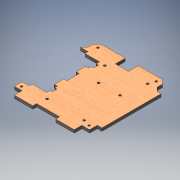
# Autodesk Inventor part: ElectronicPlate
Saved by Autodesk Inventor 2019 (Build 230136000, 136)
## iProperties
Created: 2020-12-31
Part Number: ElectronicPlate
Material: Типовые
Document SubType Name: Modeling
Designer: Professional
Density: 1 g/cm^3
Appearance: Вишневое дерево — натуральный — со слабым глянцем
Author: Professional
Autodesk Inventor part; units mm, degrees
ref_plane "YZ Plane" through (0, 0, 0) normal (1, 0, 0) x (0, 1, 0)
ref_plane "XZ Plane" through (0, 0, 0) normal (0, 1, 0) x (-1, 0, 0)
ref_plane "XY Plane" through (0, 0, 0) normal (0, 0, 1) x (1, 0, 0)
sketch "Эскиз1" plane through (0, 0, 0) normal (0, 1, 0) x (-1, 0, 0)
  line L0 (0, 0) -> (0, -96)
  line L1 (0, 0) -> (15, 0)
  line L2 (15, 0) -> (15, 5)
  line L3 (15, 5) -> (39, 5)
  line L4 (39, 5) -> (39, -5)
  line L5 (39, -5) -> (49, -5)
  line L6 (49, -5) -> (49, -15)
  line L7 (49, -15) -> (55, -15)
  line L8 (55, -15) -> (55, -92)
  line L9 (55, -92) -> (50, -92)
  line L10 (50, -92) -> (45, -97)
  line L11 (45, -97) -> (45, -104)
  line L12 (0, 0) -> (-15, 0)
  line L13 (-15, 0) -> (-15, 5)
  line L14 (-15, 5) -> (-39, 5)
  line L15 (-39, 5) -> (-39, -5)
  line L16 (-39, -5) -> (-49, -5)
  line L17 (-49, -5) -> (-49, -15)
  line L18 (-49, -15) -> (-55, -15)
  line L19 (-55, -15) -> (-55, -92)
  line L20 (-55, -92) -> (-50, -92)
  line L21 (-50, -92) -> (-45, -97)
  line L22 (-45, -97) -> (-45, -104)
  line L23 (45, -104) -> (40, -109)
  line L24 (-40, -109) -> (-45, -104)
  line L25 (40, -109) -> (8.5, -109)
  line L26 (8.5, -109) -> (8.5, -96)
  line L27 (8.5, -96) -> (0, -96)
  line L28 (-40, -109) -> (-8.5, -109)
  line L29 (-8.5, -109) -> (-8.5, -96)
  line L30 (-8.5, -96) -> (0, -96)
  point P0 (45, -109)
  point P1 (-45, -109)
  dimension "d0" = 30
  dimension "d1" = 78
  dimension "d2" = 10
  dimension "d3" = 10
  dimension "d4" = 10
  dimension "d5" = 6
  dimension "d6" = 97
  dimension "d7" = 100
  dimension "d8" = 45
  dimension "d10" = 5
  dimension "d11" = 12
  dimension "d26" = 5
  dimension "d27" = 5
  dimension "d28" = 5
  dimension "d29" = 5
  dimension "d30" = 114
  dimension "d31" = 135
  dimension "d32" = 17
  dimension "d33" = 13
  constraints: 63 end point, 13 symmetric about line, 8 perpendicular, 3 horizontal, 2 parallel, 2 point on line, 2 vertical
  measures "d0" diameter of L2 L0
  measures "d1" diameter of L4 L0
  measures "d2" distance between parallel lines of L6 L4
  measures "d3" distance between parallel lines of L5 L3
  measures "d4" distance from line of L6.end L5
  measures "d5" distance between parallel lines of L6 L8
  measures "d6" distance between parallel lines of L3 L9
  measures "d7" diameter of L9.end L0
  measures "d8" angle of L9 L10
  measures "d10" distance of L1.end L2.end
  measures "d11" distance of L10.end point (45, -109)
  measures "d26" distance of L11.end point (45, -109)
  measures "d27" distance of L23.end point (45, -109)
  measures "d28" distance of L24.start point (-45, -109)
  measures "d29" distance of L22.end point (-45, -109)
  measures "d30" distance between parallel lines of L3 L25
  measures "d31" angle of L25 L23
  measures "d32" distance between parallel lines of L29 L26
  measures "d33" distance between parallel lines of L25 L27
extrude "Выдавливание1" add sketch "Эскиз1" along normal blind 4
sketch "Эскиз2" plane through (0, 4, 0) normal (0, 1, 0) x (1, 0, 0)
  line L0 (0, 0) -> (0, 94.8396)
  line L1 (49, 5) -> (49, 15) projected
  line L2 (39, 5) -> (49, 5) projected
  line L3 (-39, -5) -> (-15, -5) projected
  line L4 (55, 15) -> (55, 92) projected
  line L5 (55, 92) -> (50, 92) projected
  line L6 (-55, 92) -> (-55, 15) projected
  line L7 (-55, 15) -> (-49, 15) projected
  point P0 (-38, 102.8)
  point P1 (38, 102.8)
  point P2 (44, 9.4)
  point P3 (-44, 9.4)
  dimension "d21" = 5
  dimension "d22" = 4.4
  dimension "d24" = 107.8
  dimension "d25" = 76
  constraints: 2 end point, 2 symmetric about line, 1 vertical
  measures "d21" distance from line of L1 point (44, 9.4)
  measures "d22" distance from line of L2 point (44, 9.4)
  measures "d24" distance from line of point (-38, 102.8) L3
  measures "d25" distance of point (38, 102.8) point (-38, 102.8)
hole "Отверстие1" at (-38, 4, -102.8) at (38, 4, -102.8) at (44, 4, -9.4) at (-44, 4, -9.4) direction (0, -1, 0) diameter 2.8 end through all
sketch "Эскиз4" plane through (0, 4, 0) normal (0, 1, 0) x (1, 0, 0)
  line L0 (-55, 92) -> (-55, 15) projected
  line L1 (-55, 88) -> (-25, 88)
  line L2 (-25, 88) -> (-25, 19)
  line L3 (-25, 19) -> (-55, 19)
  line L4 (-55, 19) -> (-55, 88)
  line L5 (-25, 88) -> (-21, 88)
  line L6 (-21, 88) -> (-21, 74)
  line L7 (-21, 74) -> (-25, 74)
  line L8 (-25, 61.5) -> (-21, 61.5)
  line L9 (-21, 61.5) -> (-21, 45.5)
  line L10 (-21, 45.5) -> (-25, 45.5)
  line L11 (-55, 53.5) -> (-25, 53.5) construction
  line L12 (-25, 19) -> (-21, 19)
  line L13 (-21, 19) -> (-21, 33)
  line L14 (-21, 33) -> (-25, 33)
  line L15 (-25, 33) -> (-25, 19)
  line L16 (-50, 92) -> (-55, 92) projected
  line L17 (-55, 92) -> (-40, 92)
  line L18 (-40, 92) -> (-40, 88)
  line L19 (-40, 88) -> (-55, 88)
  line L20 (-55, 88) -> (-55, 92)
  line L21 (-55, 15) -> (-40, 15)
  line L22 (-40, 15) -> (-40, 19)
  line L23 (-40, 19) -> (-55, 19)
  line L24 (-55, 19) -> (-55, 15)
  line L25 (-21, 23.5) -> (-18, 23.5)
  line L26 (-18, 23.5) -> (-18, 29.5)
  line L27 (-18, 29.5) -> (-21, 29.5)
  line L28 (-21, 29.5) -> (-21, 23.5)
  line L29 (-21, 77.5) -> (-18, 77.5)
  line L30 (-18, 77.5) -> (-18, 83.5)
  line L31 (-18, 83.5) -> (-21, 83.5)
  line L32 (-21, 83.5) -> (-21, 77.5)
  point P0 (0, 0)
  point P1 (-21, 53.5)
  point P2 (-18, 80.5)
  point P3 (-18, 26.5)
  dimension "d48" = 30
  dimension "d50" = 14
  dimension "d51" = 16
  dimension "d52" = 4
  dimension "d55" = 4
  dimension "d56" = 15
  dimension "d57" = 54
  dimension "d58" = 6
  dimension "d59" = 3
  constraints: 62 end point, 11 parallel, 9 point on line, 8 midpoint, 8 perpendicular, 5 horizontal, 3 symmetric about line, 2 collinear, 2 vertical alignment, 1 horizontal alignment, 1 other
  measures "d48" distance between parallel lines of L0 L2
  measures "d50" distance of L5.end L6.end
  measures "d51" distance between parallel lines of L8 L10
  measures "d52" distance between parallel lines of L2 L6
  measures "d55" distance between parallel lines of L17 L1
  measures "d56" distance between parallel lines of L2 L18
  measures "d57" distance of point (-18, 26.5) point (-18, 80.5)
  measures "d58" distance between parallel lines of L31 L29
  measures "d59" distance between parallel lines of L6 L30
extrude "Выдавливание2" cut sketch "Эскиз4" against normal through all
sketch "Эскиз5" plane through (0, 4, 0) normal (0, 1, 0) x (1, 0, 0)
  line L0 (55, 15) -> (55, 92) projected
  line L1 (15, -5) -> (39, -5) projected
  point P0 (0, 0)
  point P1 (-13.3, 12)
  point P2 (35, 12)
  point P3 (35, 94.6)
  point P4 (-13.3, 87.1)
  point P5 (2.1, 63.6)
  point P6 (30.1, 63.6)
  dimension "d67" = 48.3
  dimension "d68" = 82.6
  dimension "d69" = 75.1
  dimension "d70" = 28
  dimension "d71" = 4.9
  dimension "d72" = 20
  dimension "d73" = 17
  dimension "d74" = 51.6
  constraints: 2 horizontal alignment, 2 vertical alignment
  measures "d67" distance of point (-13.3, 12) point (35, 12)
  measures "d68" distance of point (35, 94.6) point (35, 12)
  measures "d69" distance of point (-13.3, 87.1) point (-13.3, 12)
  measures "d70" distance of point (30.1, 63.6) point (2.1, 63.6)
  measures "d71" horizontal distance of point (35, 12) point (30.1, 63.6)
  measures "d72" distance from line of L0 point (35, 12)
  measures "d73" distance from line of L1 point (35, 12)
  measures "d74" vertical distance of point (35, 12) point (30.1, 63.6)
hole "Отверстие2" at (-13.3, 4, -12) at (35, 4, -12) at (35, 4, -94.6) at (-13.3, 4, -87.1) at (2.1, 4, -63.6) at (30.1, 4, -63.6) direction (0, -1, 0) diameter 3 end through all
equation "\"d27\" = d26"
equation "\"d28\" = d26"
equation "\"d29\" = d28"
